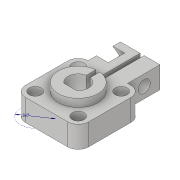
# Autodesk Inventor part: clamping hub 1_4 D b
Saved by Autodesk Inventor 2020 (Build 240168000, 168)
## iProperties
Created: 2019-10-18
Part Number: clamping hub 1_4 D b
Material: Generic
Document SubType Name: Modeling
Designer: ball
Density: 1 g/cm^3
Appearance: Default
Author: ball
Autodesk Inventor part; units mm, degrees
ref_plane "YZ Plane" through (0, 0, 0) normal (1, 0, 0) x (0, 1, 0)
ref_plane "XZ Plane" through (0, 0, 0) normal (0, 1, 0) x (-1, 0, 0)
ref_plane "XY Plane" through (0, 0, 0) normal (0, 0, 1) x (1, 0, 0)
sketch "Sketch1" plane through (0, 0, 0) normal (0, 1, 0) x (-1, 0, 0)
  line L0 (-10.16, 10.16) -> (10.16, 10.16)
  line L1 (10.16, 10.16) -> (10.16, -10.16)
  line L2 (-10.16, -10.16) -> (-10.16, 10.16)
  circle A0 centre (6.9088, -6.9148) radius 1.9304
  circle A1 centre (6.9088, 6.9088) radius 1.9304
  circle A2 centre (-6.9088, 6.9088) radius 1.9304
  circle A3 centre (-6.9088, -6.9148) radius 1.9304
  line L3 (-5.715, -10.16) -> (-5.715, -20.574)
  line L4 (-5.715, -20.574) -> (6.985, -20.574)
  line L5 (6.985, -20.574) -> (6.985, -10.16)
  line L6 (10.16, -10.16) -> (6.985, -10.16)
  line L7 (-5.715, -10.16) -> (-10.16, -10.16)
  point P0 (0, 0)
  dimension "d0" = 20.32
  dimension "d2" = 10.16
  dimension "d3" = 10.16
  dimension "d4" = 3.8608
  dimension "d5" = 6.9148
  dimension "d6" = 6.9088
  dimension "d7" = 3.8608
  dimension "d8" = 6.9088
  dimension "d9" = 6.9088
  dimension "d10" = 3.8608
  dimension "d11" = 6.9088
  dimension "d12" = 6.9088
  dimension "d13" = 3.8608
  dimension "d14" = 12.7
  dimension "d16" = 6.985
  constraints: 16 end point, 4 centre point, 4 parallel, 1 horizontal, 1 perpendicular
  measures "d0" distance of L1.end L2.start
  measures "d2" distance from line of L0 point (0, 0)
  measures "d3" distance from line of L1 point (0, 0)
  measures "d4" diameter of A0
  measures "d5" vertical distance of A0.centre point (0, 0)
  measures "d6" horizontal distance of A0.centre point (0, 0)
  measures "d7" diameter of A1
  measures "d8" horizontal distance of point (0, 0) A1.centre
  measures "d9" horizontal distance of point (0, 0) A1.centre
  measures "d10" diameter of A2
  measures "d11" horizontal distance of point (0, 0) A2.centre
  measures "d12" horizontal distance of A2.centre point (0, 0)
  measures "d13" diameter of A3
  measures "d14" distance of L4.end L3.end
  measures "d16" distance from line of L5 point (0, 0)
extrude "Extrusion1" add sketch "Sketch1" along normal blind 6.985
sketch "Sketch2" plane through (-6.985, 0, -20.574) normal (-1, 0, 0) x (0, 0, 1)
  circle A0 centre (5.08, 3.4925) radius 4.6609 construction
  line L0 (10.414, 0) -> (0, 0) projected
  line L1 (0, 0) -> (0, 6.985) projected
  line L2 (9.7409, 3.4925) -> (7.4105, -0.544)
  line L3 (7.4105, -0.544) -> (2.7496, -0.544)
  line L4 (2.7496, -0.544) -> (0.4191, 3.4925)
  line L5 (0.4191, 3.4925) -> (2.7495, 7.529)
  line L6 (2.7495, 7.529) -> (7.4104, 7.529)
  line L7 (7.4104, 7.529) -> (9.7409, 3.4925)
  point P0 (20.574, 0)
  dimension "d19" = 9.3218
  dimension "d20" = 3.4925
  dimension "d21" = 5.08
  constraints: 12 end point, 1 coincident, 1 horizontal alignment, 15 other
  measures "d20" distance from line of L0 point (5.08, 3.493)
  measures "d21" distance from line of L1 point (5.08, 3.493)
extrude "Extrusion2" cut sketch "Sketch2" against normal blind 3.81
sketch "Sketch3" plane through (5.715, 0, -10.16) normal (1, 0, 0) x (0, 0, -1)
  circle A0 centre (5.334, 3.4925) radius 1.9304
  line L0 (10.414, 0) -> (10.414, 6.985) projected
  line L1 (0, 6.985) -> (10.414, 6.985) projected
  point P0 (-10.16, 0)
  dimension "d24" = 3.8608
  dimension "d25" = 5.08
  dimension "d26" = 3.4925
  constraints: 1 centre point
  measures "d24" diameter of A0
  measures "d25" distance from line of L0 A0.centre
  measures "d26" distance from line of L1 A0.centre
extrude "Extrusion3" cut sketch "Sketch3" against normal through all
sketch "Sketch4" plane through (0, 6.985, 0) normal (0, 1, 0) x (1, 0, 0)
  circle A0 centre (0, 0) radius 6.35
  dimension "d29" = 12.7
  constraints: 1 centre point, 1 coincident
  measures "d29" diameter of A0
extrude "Extrusion4" add sketch "Sketch4" along normal blind 2.54
sketch "Sketch5" plane through (0, 9.525, 0) normal (0, 1, 0) x (1, 0, 0)
  arc A0 (2.0472, -2.5908) -> (-2.0472, -2.5908) centre (0, 0) ccw
  line L0 (-2.0472, -2.5908) -> (2.0472, -2.5908)
  dimension "d32" = 6.604
  dimension "d33" = 2.5908
  constraints: 2 end point, 2 point on circle, 1 centre point, 1 coincident, 1 horizontal
  measures "d32" diameter of A0
  measures "d33" distance from line of L0 point (0, 0)
fillet "Fillet1" radius 3.3782 4 edges at (10.16, 3.4925, 10.16) (10.16, 3.4925, -10.16) (-10.16, 3.4925, 10.16) (-10.16, 3.4925, -10.16)
extrude "Extrusion5" cut sketch "Sketch5" against normal through all
sketch "Sketch6" plane through (0, 9.525, 0) normal (0, 1, 0) x (1, 0, 0)
  line L0 (-6.985, 20.574) -> (5.715, 20.574) projected
  line L1 (0.635, 0) -> (0.635, 20.574)
  line L2 (0.635, 20.574) -> (-0.635, 20.574)
  line L3 (-0.635, 20.574) -> (-0.635, 0)
  line L4 (-0.635, -20.574) -> (0.635, 20.574) construction
  line L5 (0.635, -20.574) -> (-0.635, 20.574) construction
  line L6 (-0.635, 0) -> (0.635, 0)
  point P0 (0, 0)
  dimension "d37" = 1.27
  constraints: 12 end point, 2 midpoint, 1 parallel, 1 point on line
  measures "d37" distance of L2.end L1.end
extrude "Extrusion6" cut sketch "Sketch6" against normal through all
sketch "Sketch7" plane through (0, 0, 0) normal (0, -1, 0) x (1, 0, 0)
  circle A0 centre (-6.9088, 6.9088) radius 1.9304 construction
  circle A1 centre (-6.9088, 6.9088) radius 4.6609 construction
  point P0 (0, 0)
  dimension "d40" = 9.3218
  constraints: 1 centre point, 1 coincident
  measures "d40" diameter of A1
body "Solid1"
